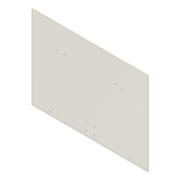
# Autodesk Inventor part: GE-12012
Saved by Autodesk Inventor 2012 (Build 160160000, 160)
## iProperties
Created: 2011-05-25
Part Number: GE-12012
Document SubType Name: Modeling
Designer: dfoster
Density: 1 g/cm^3
Description: Backboard, Top
Material: Default
Title: Backboard, Top
Author: dfoster
Autodesk Inventor part; units mm, degrees
ref_plane "YZ Plane" through (0, 0, 0) normal (1, 0, 0) x (0, 1, 0)
ref_plane "XZ Plane" through (0, 0, 0) normal (0, 1, 0) x (-1, 0, 0)
ref_plane "XY Plane" through (0, 0, 0) normal (0, 0, 1) x (1, 0, 0)
sketch "Sketch1" plane through (0, 0, 0) normal (0, 0, 1) x (1, 0, 0)
  line L0 (0, 0) -> (1117.6, 0)
  line L1 (1117.6, 0) -> (1117.6, 800.1)
  line L2 (1117.6, 800.1) -> (0, 800.1)
  line L3 (0, 800.1) -> (0, 0)
  dimension "d0" = 1117.6
  dimension "d1" = 800.1
  constraints: 8 end point, 2 parallel, 1 horizontal, 1 perpendicular
  measures "d0" distance of L1.end L2.end
  measures "d1" distance of L2.end L0.start
extrude "Extrusion1" add sketch "Sketch1" along normal blind 12.7
hole "Hole1" at (518.3188, 41.275, 12.7) direction (0, 0, -1) diameter 6.731 end through all
pattern_linear "Rectangular Pattern1" count 2 spacing 66.675 along (0, 1, 0) count 2 spacing 80.9625 along (1, 0, 0) of "Hole1"
hole "Hole2" at (241.3, 574.675, 12.7) direction (0, 0, -1) diameter 6.731 depth 25.4 tip angle 118 countersink diameter 12.7 countersink angle 82
pattern_linear "Rectangular Pattern2" count 2 spacing 76.2 along (1, 0, 0) of "Hole2"
hole "Hole3" at (876.3, 574.675, 12.7) direction (0, 0, -1) diameter 6.731 depth 25.4 tip angle 118 countersink diameter 12.7 countersink angle 82
pattern_linear "Rectangular Pattern3" count 2 spacing 76.2 along (-1, 0, 0) of "Hole3"
hole "Hole4" at (174.625, 28.575, 12.7) direction (0, 0, -1) diameter 6.731 depth 25.4 tip angle 118 countersink diameter 12.7 countersink angle 82
hole "Hole5" at (942.975, 28.575, 12.7) direction (0, 0, -1) diameter 6.731 depth 25.4 tip angle 118 countersink diameter 12.7 countersink angle 82
body "Solid1"
